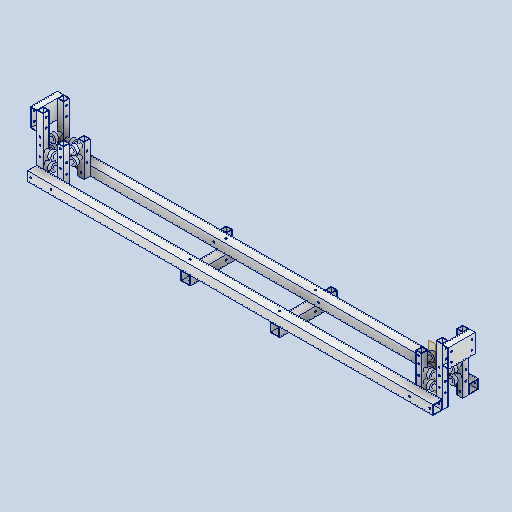
# Autodesk Inventor part: RZvector-Srunit-v3-ASP-Base
Saved by Autodesk Inventor 2025.2 (Build 292293000, 293)
## iProperties
Created: 2024-04-13
Part Number: RZvector-Srunit-v3-ASP-Base
Material: アルミニウム 6061
Document SubType Name: Modeling
Designer: haruy
Density: 2.7 g/cm^3
Appearance: アルミニウム - フラット
Author: haruy
Autodesk Inventor part; units mm, degrees
ref_plane "YZ Plane" through (0, 0, 0) normal (1, 0, 0) x (0, 1, 0)
ref_plane "XZ Plane" through (0, 0, 0) normal (0, 1, 0) x (-1, 0, 0)
ref_plane "XY Plane" through (0, 0, 0) normal (0, 0, 1) x (1, 0, 0)
derived "RZvector-Srunit-v2-Sketch-Base.ipt"
sketch "正面から" plane through (0, 0, 0) normal (0, 0, 1) x (1, 0, 0)
  line L0 (0, 0) -> (20, 0)
  line L1 (20, 0) -> (20, 80)
  line L2 (20, 80) -> (0, 80)
  line L3 (0, 80) -> (0, 0)
  line L4 (21.5, 92) -> (31.5, 92)
  line L5 (31.5, 92) -> (31.5, 0)
  line L6 (31.5, 0) -> (21.5, 0)
  line L7 (21.5, 0) -> (21.5, 92)
  line L8 (-11.5, 62) -> (-1.5, 62)
  line L9 (-1.5, 62) -> (-1.5, 0)
  line L10 (-1.5, 0) -> (-11.5, 0)
  line L11 (-11.5, 0) -> (-11.5, 62)
  line L12 (-1.5, 24.5) -> (21.5, 24.5)
  line L13 (21.5, 24.5) -> (21.5, 18.5)
  line L14 (21.5, 18.5) -> (-1.5, 18.5)
  line L15 (-1.5, 18.5) -> (-1.5, 24.5)
  line L16 (7.5, 28) -> (12.5, 28)
  line L17 (12.5, 28) -> (12.5, 15)
  line L18 (12.5, 15) -> (7.5, 15)
  line L19 (7.5, 15) -> (7.5, 28)
  circle A0 centre (26.5, 29.5) radius 3
  line L20 (31.5, 15) -> (-189.7387, 15)
  line L21 (-189.7387, 15) -> (-189.7387, 0)
  line L22 (-189.7387, 0) -> (31.5, 0)
  line L23 (31.5, 0) -> (31.5, 15)
  line L24 (31.5, 92) -> (41.5, 92)
  line L25 (41.5, 92) -> (41.5, 62)
  line L26 (41.5, 62) -> (31.5, 62)
  line L27 (31.5, 62) -> (31.5, 92)
  circle A1 centre (26.5, 29.5) radius 6.5
  circle A2 centre (-6.5, 29.5) radius 6.5
  line L28 (21.5, 23) -> (31.5, 23)
  line L29 (21.5, 20) -> (31.5, 20)
  circle A3 centre (26.5, 29.5) radius 1.5
  circle A4 centre (-6.5, 29.5) radius 3
  circle A5 centre (-6.5, 29.5) radius 1.5
  line L30 (-1.5, 40.5) -> (21.5, 40.5)
  line L31 (21.5, 40.5) -> (21.5, 34.5)
  line L32 (21.5, 34.5) -> (-1.5, 34.5)
  line L33 (-1.5, 34.5) -> (-1.5, 40.5)
  line L34 (7.5, 44) -> (12.5, 44)
  line L35 (12.5, 44) -> (12.5, 31)
  line L36 (12.5, 31) -> (7.5, 31)
  line L37 (7.5, 31) -> (7.5, 44)
  circle A6 centre (-6.5, 45.5) radius 6.5
  circle A7 centre (-6.5, 45.5) radius 3
  circle A8 centre (-6.5, 45.5) radius 1.5
  line L38 (-11.5, 62) -> (31.5, 62)
  line L39 (31.5, 62) -> (31.5, 52)
  line L40 (31.5, 52) -> (-11.5, 52)
  line L41 (-11.5, 52) -> (-11.5, 62)
  circle A9 centre (26.5, 45.5) radius 6.5
  circle A10 centre (26.5, 45.5) radius 3
  circle A11 centre (26.5, 45.5) radius 1.5
  line L42 (31.5, 47) -> (31.5, 62)
  line L43 (-145, 64.5) -> (31.5, 64.5)
  line L44 (31.5, 64.5) -> (31.5, 49.5)
  line L45 (31.5, 49.5) -> (-145, 49.5)
  line L46 (-145, 49.5) -> (-145, 64.5)
  point P0 (-6.5, 7.5)
  point P1 (26.5, 7.5)
  point P2 (-6.5, 57)
  point P3 (10, 57)
  point P4 (26.5, 57)
  point P5 (-1.5, 52)
  point P6 (-1.5, 62)
  point P7 (-135, 56.75)
  point P8 (-1.5, 49.5)
  point P9 (-1.5, 49.6533)
  point P10 (-1.3765, 49.5)
  dimension "d1" = 7.5
  dimension "d2" = 7.5
  dimension "d3" = 5
  dimension "d4" = 5
  dimension "d5" = 5
  dimension "d6" = 5
  dimension "d7" = 10
  dimension "d8" = 5
  dimension "d9" = 5
  dimension "d10" = 5
  dimension "d90" = 176.5
  dimension "d91" = 15
  dimension "d92" = 2.5
  dimension "d93" = 0
  dimension "d94" = 7.25
  dimension "d95" = 10
  measures "d1" distance from line of point (-6.5, 7.5) L10
  measures "d2" distance from line of point (26.5, 7.5) L6
  measures "d3" distance from line of point (-6.5, 7.5) L9
  measures "d4" distance from line of point (26.5, 7.5) L7
  measures "d5" distance from line of point (-6.5, 57) L8
  measures "d6" distance from line of point (-6.5, 57) L9
  measures "d7" distance from line of point (10, 57) L3
  measures "d8" distance from line of point (10, 57) L40
  measures "d9" distance from line of L38 point (26.5, 57)
  measures "d10" distance from line of point (26.5, 57) L5
  measures "d90" distance of L44.end L45.end
  measures "d91" distance of L43.end L44.end
  measures "d92" distance between parallel lines of L8 L43
  measures "d93" distance between parallel lines of L5 L44
  measures "d94" distance from line of point (-135, 56.75) L45
  measures "d95" distance from line of L46 point (-135, 56.75)
sketch "横から" plane through (0, 0, 0) normal (1, 0, 0) x (0, 1, 0)
  line L0 (0, 0) -> (200, 0)
  line L1 (200, 0) -> (200, -20)
  line L2 (200, -20) -> (0, -20)
  line L3 (0, -20) -> (0, 0)
  circle A0 centre (21.5, 6.5) radius 6.5
  circle A1 centre (21.5, -26.5) radius 6.5
  line L4 (15, 26.5) -> (0, 26.5)
  line L5 (0, 26.5) -> (0, 11.5)
  line L6 (0, 11.5) -> (15, 11.5)
  line L7 (15, 11.5) -> (15, 26.5)
  line L8 (15, -31.5) -> (0, -31.5)
  line L9 (0, -31.5) -> (0, -46.5)
  line L10 (0, -46.5) -> (15, -46.5)
  line L11 (15, -46.5) -> (15, -31.5)
  line L12 (62, 11.5) -> (0, 11.5)
  line L13 (0, 11.5) -> (0, 1.5)
  line L14 (0, 1.5) -> (62, 1.5)
  line L15 (62, 1.5) -> (62, 11.5)
  line L16 (62, -21.5) -> (0, -21.5)
  line L17 (0, -21.5) -> (0, -31.5)
  line L18 (0, -31.5) -> (62, -31.5)
  line L19 (62, -31.5) -> (62, -21.5)
  line L20 (36, -7.5) -> (23, -7.5)
  line L21 (23, -7.5) -> (23, -12.5)
  line L22 (23, -12.5) -> (36, -12.5)
  line L23 (36, -12.5) -> (36, -7.5)
  line L24 (92, 11.5) -> (62, 11.5)
  line L25 (62, 11.5) -> (62, -31.5)
  line L26 (62, -31.5) -> (92, -31.5)
  line L27 (92, -31.5) -> (92, 11.5)
  circle A2 centre (37.5, 6.5) radius 6.5
  circle A3 centre (37.5, -26.5) radius 6.5
  line L28 (52, -7.5) -> (39, -7.5)
  line L29 (39, -7.5) -> (39, -12.5)
  line L30 (39, -12.5) -> (52, -12.5)
  line L31 (52, -12.5) -> (52, -7.5)
  point P0 (62, -26.5)
extrude "押し出し1" add sketch "正面から" along normal blind 10 contours L10 L11 L20 L9 | L20 L11 A2 L9 | L11 A2 L9 | A2 L11 A6 L9 | L11 L45 L9 A6 | L11 A6 L9 L45 | L11 L40 A6 | A6 L40 L9 | L11 L8 L9 L40 | A4 | A5 | A7 | A8
extrude "押し出し2" add sketch "正面から" along normal blind 10 separate body contours L7 L20 L5 L6 | L7 L29 L5 L20 | L7 A1 L28 | L7 L28 L5 L29 | A1 L5 L7 | L7 A9 L5 A1 | L28 A1 L5 | A9 L7 L45 L5 | A9 L5 L45 L7 | L7 L40 A9 | A9 L40 L5 | L7 L38 L5 L40 | L7 L43 L5 L38 | L7 L4 L5 L43 | A0 | A3 | A10 | A11
ref_plane "作業平面1" through (-1.5, 0, -23) normal (0, 0, -1) x (-1, 0, 0)
extrude "押し出し3" add sketch "正面から" against normal blind 10 from surface at -23 separate body contours L10 L11 L20 L9 | L20 L11 A2 L9 | L11 A2 L9 | A2 L11 A6 L9 | L11 L45 L9 A6 | L11 A6 L9 L45 | L11 L40 A6 | A6 L40 L9 | A4 | A5 | A7 | A8
extrude "押し出し4" add sketch "正面から" against normal blind 10 from surface at -23 separate body contours L7 L20 L5 L6 | L7 L29 L5 L20 | L7 A1 L28 | L7 L28 L5 L29 | A1 L5 L7 | L7 A9 L5 A1 | L28 A1 L5 | A9 L7 L45 L5 | A9 L5 L45 L7 | L7 L40 A9 | A9 L40 L5 | L7 L38 L5 L40 | L7 L43 L5 L38 | L7 L4 L5 L43 | A0 | A3 | A10 | A11
ref_plane "作業平面2" through (-11.5, 0, 10) normal (0, 0, 1) x (1, 0, 0)
extrude "押し出し5" add sketch "正面から" along normal blind 15 from surface at 10 separate body contours L45 A6 L11 | L11 A6 L9 L45 | L45 L46 L43 L3 L38 L8 L11 A6 | L45 A6 L9 L40 L3 | L3 L40 L1 L45 | L45 L9 A6 | L11 L40 A6 | L1 L40 L7 A9 L45 | A9 L7 L45 | L40 L9 L38 L3 | L3 L38 L1 L40 | A6 L40 L9 | L11 L8 L9 L40 | L1 L38 L7 L40 | A9 L5 L45 L7 | L7 L40 A9 | A9 L40 L5 | L3 L43 L1 L38 | L1 L43 L7 L38 | L7 L38 L5 L40 | L7 L43 L5 L38 picked at (-11.5139, 49.5853) picked at (-6.5, 50.3333) picked at (-1.4861, 49.5853) picked at (21.4861, 49.5853) picked at (26.5, 50.3333)
sketch "スケッチ3" plane through (31.5, 0, 0) normal (1, 0, 0) x (0, 0, -1)
  line L0 (-10, 92) -> (-10, 0) projected
  line L1 (-10, 92) -> (33, 92)
  line L2 (33, 92) -> (33, 62)
  line L3 (33, 62) -> (-10, 62)
  line L4 (-10, 62) -> (-10, 92)
  point P0 (0, 0)
  dimension "d23" = 43
  dimension "d24" = 30
  constraints: 8 end point, 2 parallel, 1 horizontal, 1 perpendicular
  measures "d23" distance of L2.end L3.end
  measures "d24" distance of L1.end L2.end
extrude "押し出し6" add sketch "スケッチ3" along normal blind 10 separate body
shell "シェル1" thickness 1 removed faces 11 at (-4.8333, 52, -26.3333) at (-8.1667, 0, -26.3333) at (24.8333, 0, -26.3333) at (-8.1667, 0, 3.3333) at (24.8333, 0, 3.3333) at (31.5, 54.5, 20) at (28.1667, 92, 6.6667) at (28.1667, 92, -26.3333) at (38.1667, 72, 10) at (34.8333, 72, -33) at (-4.8333, 62, 3.3333) bodies 3 4 1 2 5 6
hole "穴1" at (-6.5, 7.5, 0) at (26.5, 7.5, 0) at (-6.5, 57, 0) at (10, 57, 0) at (26.5, 57, 0) at (26.5, 29.5, 0) at (-6.5, 29.5, 0) at (-6.5, 45.5, 0) at (26.5, 45.5, 0) at (-135, 56.75, 0) direction (0, 0, 1) diameter 3 end through all both bodies 2 1 5 3
hole "穴2" at (26.5, 45.5, 0) at (26.5, 29.5, 0) at (26.5, 7.5, 0) direction (0, 0, -1) diameter 3 end through all bodies 4
sketch "スケッチ4" plane through (41.5, 0, 0) normal (1, 0, 0) x (0, 0, -1)
  line L0 (-10, 92) -> (-10, 62) projected
  line L1 (33, 62) -> (33, 92) projected
  line L2 (33, 92) -> (-10, 92) projected
  line L3 (0, 0) -> (-10, 0) projected
  line L4 (33, 0) -> (23, 0) projected
  line L5 (-10, 0) -> (-10, 92) projected
  line L6 (23, 0) -> (23, 92) projected
  line L7 (-10, 62) -> (33, 62) projected
  point P0 (-5, 84.5)
  point P1 (28, 84.5)
  point P2 (-5, 21.5)
  point P3 (-5, 37.5)
  point P4 (28, 37.5)
  point P5 (28, 21.5)
  point P6 (-5, 69.5)
  point P7 (28, 69.5)
  dimension "d42" = 5
  dimension "d43" = 5
  dimension "d44" = 7.5
  dimension "d45" = 7.5
  dimension "d46" = 21.5
  dimension "d47" = 21.5
  dimension "d48" = 16
  dimension "d49" = 16
  dimension "d50" = 5
  dimension "d51" = 5
  dimension "d52" = 5
  dimension "d53" = 5
  dimension "d84" = 5
  dimension "d85" = 5
  dimension "d86" = 7.5
  dimension "d87" = 7.5
  measures "d42" distance from line of point (-5, 84.5) L0
  measures "d43" distance from line of L1 point (28, 84.5)
  measures "d44" distance from line of point (-5, 84.5) L2
  measures "d45" distance from line of L2 point (28, 84.5)
  measures "d46" distance from line of point (-5, 21.5) L3
  measures "d47" distance from line of point (28, 21.5) L4
  measures "d48" distance of point (-5, 37.5) point (-5, 21.5)
  measures "d49" distance of point (28, 37.5) point (28, 21.5)
  measures "d50" distance from line of point (-5, 21.5) L5
  measures "d51" distance from line of point (-5, 37.5) L5
  measures "d52" distance from line of point (28, 21.5) L6
  measures "d53" distance from line of point (28, 37.5) L6
  measures "d84" distance from line of L0 point (-5, 69.5)
  measures "d85" distance from line of L1 point (28, 69.5)
  measures "d86" distance from line of point (-5, 69.5) L7
  measures "d87" distance from line of point (28, 69.5) L7
hole "穴3" at (41.5, 84.5, 5) at (41.5, 84.5, -28) at (41.5, 21.5, 5) at (41.5, 37.5, 5) at (41.5, 37.5, -28) at (41.5, 21.5, -28) at (41.5, 69.5, 5) at (41.5, 69.5, -28) direction (-1, 0, 0) diameter 3 end through all bodies 6 2 4 1 3
extrude "押し出し7" add sketch "正面から" against normal up to surface (23 mm away) separate body contours A0 | A4 | A7 | A10
sketch "スケッチ5" plane through (21.5, 0, -33) normal (-1, 0, 0) x (0, 0, 1)
  circle A0 centre (5, 37.5) radius 1.5 projected
  circle A1 centre (5, 37.5) radius 3
  circle A2 centre (5, 37.5) radius 1.5
  circle A3 centre (5, 21.5) radius 1.5 projected
  circle A4 centre (5, 21.5) radius 3
  circle A5 centre (5, 21.5) radius 1.5
  circle A6 centre (38, 37.5) radius 1.5 projected
  circle A7 centre (38, 37.5) radius 3
  circle A8 centre (38, 21.5) radius 1.5 projected
  circle A9 centre (38, 21.5) radius 3
  circle A10 centre (38, 21.5) radius 1.5
  circle A11 centre (38, 37.5) radius 1.5
  circle A12 centre (5, 37.5) radius 6.5
  circle A13 centre (5, 21.5) radius 6.5
  circle A14 centre (38, 21.5) radius 6.5
  circle A15 centre (38, 37.5) radius 6.5
  point P0 (33, 0)
  dimension "d63" = 6
  dimension "d64" = 3
  dimension "d65" = 6
  dimension "d66" = 3
  dimension "d67" = 6
  dimension "d68" = 6
  dimension "d69" = 3
  dimension "d70" = 3
  dimension "d76" = 13
  dimension "d77" = 13
  dimension "d78" = 13
  dimension "d79" = 13
  constraints: 12 centre point, 12 coincident
  measures "d63" diameter of A1
  measures "d64" diameter of A2
  measures "d65" diameter of A4
  measures "d66" diameter of A5
  measures "d67" diameter of A7
  measures "d68" diameter of A9
  measures "d69" diameter of A10
  measures "d70" diameter of A11
  measures "d76" diameter of A12
  measures "d77" diameter of A13
  measures "d78" diameter of A14
  measures "d79" diameter of A15
extrude "押し出し8" add sketch "スケッチ5" along normal up to surface (23 mm away) separate body contours A1 | A4 | A7 | A9
ref_plane "作業平面3" through (-1.5, 0, -11.5) normal (0, 0, -1) x (-1, 0, 0)
extrude "押し出し9" add sketch "正面から" along normal mid plane 5 from surface at -11.5 separate body contours A2 L9 | A2 L11 | L11 A2 L9 | A1 L7 | A1 L5 L7 | A6 L45 L11 | L11 L45 L9 A6 | A1 L5 | A6 L9 L45 | L45 A6 L11 | L11 A6 L9 L45 | A9 L45 L7 | A9 L7 L45 L5 | L5 A9 | L45 L9 A6 | A9 L7 L45 | A9 L5 L45 L7
ref_plane "作業平面4" through (10, 0, 0) normal (-1, 0, 0) x (0, 0, 1)
extrude "押し出し10" add sketch "スケッチ5" along normal mid plane 5 from surface at 11.5 separate body contours A12 | A13 | A14 | A15
ref_plane "作業平面5" through (-295, 0, -33) normal (-1, 0, 0) x (0, 0, 1)
mirror "ミラー1" about plane through (-295, 0, -33) normal (-1, 0, 0) bodies 1 2 3 4 5 6 7 8 9 10 separate body
sketch "スケッチ6" plane through (31.5, 0, 0) normal (1, 0, 0) x (0, 0, -1)
  line L0 (-10, 92) -> (-10, 0) projected
  line L1 (-10, 0) -> (-25, 0)
  line L2 (-25, 0) -> (-25, 15)
  line L3 (-25, 15) -> (-10, 15)
  line L4 (-10, 15) -> (-10, 0)
  line L5 (-11, 14) -> (-24, 14)
  line L6 (-24, 14) -> (-24, 1)
  line L7 (-24, 1) -> (-11, 1)
  line L8 (-11, 1) -> (-11, 14)
  point P0 (0, 0)
  dimension "d96" = 15
  dimension "d97" = 15
  dimension "d98" = 1
  constraints: 16 end point, 4 parallel, 2 perpendicular, 1 horizontal, 3 other
  measures "d96" distance of L2.end L3.end
  measures "d97" distance of L1.end L2.end
  measures "d98" distance between parallel lines of L3 L5
extrude "押し出し11" add sketch "スケッチ6" against normal up to surface (653 mm away) separate body
sketch "スケッチ7" plane through (31.5, 0, 25) normal (0, 0, 1) x (1, 0, 0)
  circle A0 centre (-5, 7.5) radius 1.5 projected
  circle A1 centre (-38, 7.5) radius 1.5 projected
  circle A2 centre (-648, 7.5) radius 1.5 projected
  circle A3 centre (-615, 7.5) radius 1.5 projected
  point P0 (-31.5, 0)
  constraints: 4 coincident
hole "穴4" at (26.5, 7.5, 25) at (-6.5, 7.5, 25) at (-616.5, 7.5, 25) at (-583.5, 7.5, 25) direction (0, 0, -1) diameter 3 end through all bodies 21
sketch "スケッチ8" plane through (31.5, 15, 25) normal (0, 1, 0) x (1, 0, 0)
  line L0 (0, 0) -> (-653, 0) projected
  line L1 (-326.5, 0) -> (-326.5, 15)
  line L2 (0, 15) -> (-653, 15) projected
  line L3 (-274, 0) -> (-294, 0)
  line L4 (-294, 0) -> (-294, 15)
  line L5 (-294, 15) -> (-274, 15)
  line L6 (-274, 15) -> (-274, 0)
  line L7 (-264, 15) -> (-264, 0)
  line L8 (-264, 0) -> (-262, 0)
  line L9 (-262, 0) -> (-262, 15)
  line L10 (-262, 15) -> (-264, 15)
  line L11 (-264, 15) -> (-264, 0)
  point P0 (-31.5, 25)
  point P1 (-254.5, 7.5)
  point P2 (-398.5, 7.5)
  dimension "d108" = 20
  dimension "d109" = 15
  dimension "d110" = 52.5
  dimension "d111" = 10
  dimension "d112" = 2
  dimension "d113" = 15
  dimension "d114" = 7.5
  dimension "d115" = 7.5
  constraints: 20 end point, 4 parallel, 3 perpendicular, 3 point on line, 2 horizontal, 2 midpoint, 1 symmetric about line
  measures "d108" distance of L4.end L5.end
  measures "d109" distance of L3.end L4.end
  measures "d110" distance between parallel lines of L6 L1
  measures "d111" distance between parallel lines of L7 L6
  measures "d112" distance of L10.end L9.end
  measures "d113" distance of L9.end L8.end
  measures "d114" distance from line of point (-254.5, 7.5) L0
  measures "d115" distance from line of point (-254.5, 7.5) L9
hole "穴5" at (-223, 15, 17.5) at (-367, 15, 17.5) direction (0, -1, 0) diameter 3 end through all bodies 21
ref_plane "作業平面6" through (-11.5, 0, -11.5) normal (0, 0, 1) x (1, 0, 0)
mirror "ミラー2" about plane through (-11.5, 0, -11.5) normal (0, 0, 1) of "押し出し11", "穴4", "穴5" bodies 21
sketch "スケッチ9" plane through (31.5, 0, 10) normal (0, -1, 0) x (1, 0, 0)
  line L0 (0, 15) -> (-653, 15) projected
  line L1 (-406, 15) -> (-391, 15)
  line L2 (-391, 15) -> (-391, -68)
  line L3 (-391, -68) -> (-406, -68)
  line L4 (-406, -68) -> (-406, 15)
  line L5 (0, -58) -> (-653, -58) projected
  circle A0 centre (-398.5, -50.5) radius 1.5 projected
  circle A1 centre (-398.5, 7.5) radius 1.5 projected
  line L6 (-326.5, -58) -> (-326.5, 15)
  line L7 (-247, 15) -> (-262, 15)
  line L8 (-262, 15) -> (-262, -68)
  line L9 (-262, -68) -> (-247, -68)
  line L10 (-247, -68) -> (-247, 15)
  circle A2 centre (-254.5, -50.5) radius 1.5
  circle A3 centre (-254.5, 7.5) radius 1.5
  point P0 (-31.5, -10)
  point P1 (-247, 15)
  point P2 (-262, 15)
  point P3 (-391, 15)
  dimension "d124" = 15
  dimension "d126" = 10
  dimension "d127" = 7.5
  constraints: 18 end point, 6 symmetric about line, 4 coincident, 2 centre point, 2 midpoint, 2 parallel, 1 horizontal, 1 perpendicular, 1 point on line
  measures "d124" distance of L2.end L3.end
  measures "d126" distance between parallel lines of L5 L3
  measures "d127" distance from line of L4 A0.centre
extrude "押し出し13" add sketch "スケッチ9" along normal blind 15 separate body contours L10 L5 L8 L0 | L10 L9 L8 L5 | L2 L5 L4 L0 | L2 L3 L4 L5 | A0 | A1 | A2 | A3
shell "シェル2" thickness 1 removed faces 4 at (-364.5, -5, 25) at (-220.5, -5, 25) at (-225.5, -10, -58) at (-369.5, -10, -58) bodies 22
hole "穴6" at (-223, 0, 17.5) at (-223, 0, -40.5) at (-367, 0, -40.5) at (-367, 0, 17.5) direction (0, -1, 0) diameter 3 end through all bodies 22
sketch "スケッチ10" plane through (31.5, -15, 10) normal (0, -1, 0) x (1, 0, 0)
  line L0 (-247, -68) -> (-247, 15) projected
  line L1 (-247, -68) -> (-237, -68)
  line L2 (-237, -68) -> (-237, -58)
  line L3 (-237, -58) -> (-247, -58)
  line L4 (-247, -58) -> (-247, -68)
  line L5 (-406, 15) -> (-406, -68) projected
  line L6 (-406, -68) -> (-416, -68)
  line L7 (-416, -68) -> (-416, -58)
  line L8 (-416, -58) -> (-406, -58)
  line L9 (-406, -58) -> (-406, -68)
  line L10 (-238, -67) -> (-246, -67)
  line L11 (-246, -67) -> (-246, -59)
  line L12 (-246, -59) -> (-238, -59)
  line L13 (-238, -59) -> (-238, -67)
  line L14 (-415, -67) -> (-407, -67)
  line L15 (-407, -67) -> (-407, -59)
  line L16 (-407, -59) -> (-415, -59)
  line L17 (-415, -59) -> (-415, -67)
  point P0 (-31.5, -10)
  dimension "d140" = 10
  dimension "d141" = 10
  dimension "d142" = 10
  dimension "d143" = 10
  dimension "d144" = 1
  dimension "d145" = 1
  constraints: 32 end point, 8 parallel, 4 perpendicular, 2 horizontal, 6 other
  measures "d140" distance of L3.end L2.end
  measures "d141" distance of L2.end L1.end
  measures "d142" distance of L7.end L8.end
  measures "d143" distance of L6.end L7.end
  measures "d144" distance between parallel lines of L1 L10
  measures "d145" distance between parallel lines of L6 L14
extrude "押し出し14" add sketch "スケッチ10" against normal up to surface (30 mm away) separate body
sketch "スケッチ11" plane through (-205.5, -15, -58) normal (0, 0, -1) x (-1, 0, 0)
  line L0 (0, 0) -> (0, 30) projected
  line L1 (10, 30) -> (0, 30) projected
  line L2 (179, 30) -> (169, 30) projected
  line L3 (179, 0) -> (179, 30) projected
  point P0 (-205.5, 15)
  point P1 (5, 22.5)
  point P2 (174, 22.5)
  dimension "d148" = 5
  dimension "d149" = 7.5
  dimension "d150" = 7.5
  dimension "d151" = 5
  measures "d148" distance from line of point (5, 22.5) L0
  measures "d149" distance from line of L1 point (5, 22.5)
  measures "d150" distance from line of point (174, 22.5) L2
  measures "d151" distance from line of L3 point (174, 22.5)
hole "穴7" at (-210.5, 7.5, -58) at (-379.5, 7.5, -58) direction (0, 0, 1) diameter 3 depth 25 tip angle 118 bodies 23 21
sketch "スケッチ12" plane through (-205.5, -15, -48) normal (1, 0, 0) x (0, 0, -1)
  line L0 (10, 0) -> (0, 0) projected
  line L1 (10, 0) -> (10, 30) projected
  point P0 (-48, 15)
  point P1 (5, 7.5)
  dimension "d159" = 7.5
  dimension "d160" = 5
  measures "d159" distance from line of point (5, 7.5) L0
  measures "d160" distance from line of point (5, 7.5) L1
hole "穴8" at (-205.5, -7.5, -53) direction (-1, 0, 0) diameter 3 depth 179 tip angle 118 bodies 23 22
sketch "スケッチ13" plane through (-215.5, 0, 25) normal (1, 0, 0) x (0, 0, -1)
  line L0 (83, -15) -> (0, -15) projected
  line L1 (0, 0) -> (0, -15) projected
  line L2 (73, -15) -> (73, 15) projected
  point P0 (25, 0)
  point P1 (15, -7.5)
  point P2 (58, -7.5)
  dimension "d168" = 7.5
  dimension "d169" = 7.5
  dimension "d170" = 15
  dimension "d171" = 15
  measures "d168" distance from line of point (15, -7.5) L0
  measures "d169" distance from line of point (58, -7.5) L0
  measures "d170" distance from line of L1 point (15, -7.5)
  measures "d171" distance from line of point (58, -7.5) L2
hole "穴9" at (-215.5, -7.5, 10) at (-215.5, -7.5, -33) direction (-1, 0, 0) diameter 3 depth 159 tip angle 118 bodies 22
equation "\"d169\" = d168"
